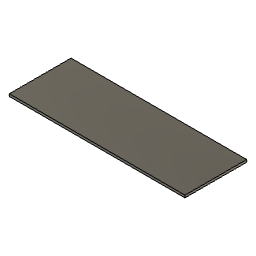
cover_front v1 (Autodesk Fusion 360 design; units mm, degrees)
Autodesk Fusion 360 part; units mm, degrees
sketch "Skizze1" plane through (0, 0, 0) normal (0, 0, 1) x (1, 0, 0)
  line L0 (74, -26) -> (-74, -26)
  line L1 (-74, -26) -> (-74, 26)
  line L2 (-74, 26) -> (74, 26)
  line L3 (74, 26) -> (74, -26)
  line L4 (74, -26) -> (-74, 26) construction
  line L5 (-74, -26) -> (74, 26) construction
  dimension "d1" = 148
  dimension "d2" = 52
  constraint horizontal L0
  constraint perpendicular L0 L1
  constraint parallel L0 L2
  constraint parallel L1 L3
  constraint coincident L4 origin
  constraint coincident L5 origin
  measures "d1" distance of L1 L3
  measures "d2" distance of L0 L2
extrude "Extrusion1" add sketch "Skizze1" along normal blind 2
